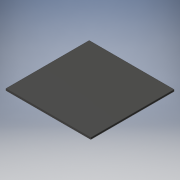
# Autodesk Inventor part: Pickup Rubber
Saved by Autodesk Inventor 2016 (Build 200138000, 138)
## iProperties
Created: 2015-11-25
Part Number: Pickup Rubber
Material: Rubber
Document SubType Name: Modeling
Designer: Julia
Density: 0.93 g/cm^3
Appearance: Rubber - Black
Author: Julia
Autodesk Inventor part; units mm, degrees
ref_plane "YZ Plane" through (0, 0, 0) normal (1, 0, 0) x (0, 1, 0)
ref_plane "XZ Plane" through (0, 0, 0) normal (0, 1, 0) x (-1, 0, 0)
ref_plane "XY Plane" through (0, 0, 0) normal (0, 0, 1) x (1, 0, 0)
sketch "Sketch1" plane through (0, 0, 0) normal (0, 1, 0) x (-1, 0, 0)
  line L0 (0, 0) -> (0, -86.36)
  line L1 (0, -86.36) -> (88.011, -86.36)
  line L2 (88.011, -86.36) -> (88.011, 0)
  line L3 (88.011, 0) -> (0, 0)
  dimension "d0" = 86.36
  dimension "d1" = 88.011
  constraints: 8 end point, 3 perpendicular, 1 vertical
  measures "d0" distance of L0.start L0.end
  measures "d1" distance of L0.end L1.end
extrude "Extrusion1" add sketch "Sketch1" along normal blind 1.8034
body "Solid1"
